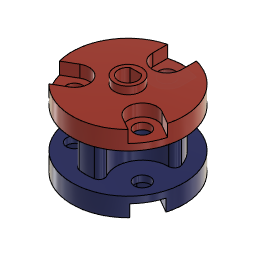
Rotor (Autodesk Fusion 360 design; units mm, degrees)
Autodesk Fusion 360 part; units mm, degrees
sketch "Sketch1" plane through (0, 0, 0) normal (0, 0, 1) x (1, 0, 0)
  circle A0 centre (0, 0) radius 15
  dimension "d1" = 30
  constraint coincident A0.centre origin
  measures "d1" diameter of A0
extrude "Extrude1" add sketch "Sketch1" along normal blind 5 contours A0 picked at (3.831549, 5.619851) makes body 1
sketch "Sketch2" plane through (0, 0, 5) normal (0, 0, 1) x (-1, 0, 0)
  circle A0 centre (0, 0) radius 15
  circle A1 centre (0, 0) radius 2.6
  circle A2 centre (0, 0) radius 3.6
  line L0 (0.004273, -1.599996) -> (2.049393, -1.599996)
  line L1 (0.004273, -1.599996) -> (-2.049393, -1.599996)
  dimension "d4" = 5.2
  dimension "d5" = 1
  constraint concentric A0 A1
  measures "d4" diameter of A1
extrude "Extrude2" add sketch "Sketch2" along normal blind 2 contours A2 picked at (-3.178319, -0.724982) bodies 1
extrude "Extrude3" cut 1 faces at (-0.716074, -0.488211, 5) along direction (0, 0, -1) blind 5 on bodies 1 bodies 1
sketch "Sketch3" plane through (0, 0, 5) normal (0, 0, 1) x (-1, 0, 0)
  circle A0 centre (0, 0) radius 15
  circle A1 centre (0, 0) radius 3.6
  arc A2 (0, -15) -> (12.990381, 7.5) centre (0, 0) ccw
  line L0 (0, 0) -> (0, -15) construction
  line L1 (0, 0) -> (12.990381, 7.5) construction
  arc A3 (-12.990381, 7.5) -> (0, -15) centre (0, 0) ccw
  line L2 (0, 0) -> (-12.990381, 7.5) construction
  line L3 (0, 0) -> (0, -15) construction
  circle A4 centre (0, -11.5) radius 3.5
  circle A5 centre (-9.959292, 5.75) radius 3.5
  line L4 (0, -11.5) -> (3.5, -11.5)
  line L5 (-3.5, -11.498985) -> (0.073703, -11.498985)
  line L6 (3.5, -11.5) -> (3.5, -14.585952)
  line L7 (-3.5, -11.5) -> (-3.5, -14.585952)
  line L8 (3.5, -11.5) -> (0, -8)
  line L9 (-3.5, -11.498985) -> (0, -8)
  arc A6 (0, -15) -> (12.990381, -7.5) centre (0, 0) ccw
  line L10 (0, 0) -> (0, -15) construction
  line L11 (0, 0) -> (12.990381, -7.5) construction
  line L12 (0, 0) -> (0, 15)
  line L13 (-8.209292, 8.781089) -> (-10.881805, 10.324065)
  circle A7 centre (-9.959292, 5.75) radius 3.5
  line L14 (-8.208413, 8.780581) -> (-9.995265, 5.685663)
  line L15 (-8.208413, 8.780581) -> (-6.928203, 4)
  line L16 (-11.709292, 2.718911) -> (-6.928203, 4)
  line L17 (-9.959292, 5.75) -> (-11.709292, 2.718911)
  line L18 (-11.709292, 2.718911) -> (-14.381805, 4.261887)
  circle A8 centre (9.959292, 5.75) radius 3.5
  line L19 (11.709292, 2.718911) -> (14.381805, 4.261887)
  line L20 (9.959292, 5.75) -> (11.709292, 2.718911)
  line L21 (11.709292, 2.718911) -> (6.928203, 4)
  line L22 (8.208413, 8.780581) -> (6.928203, 4)
  line L23 (8.208413, 8.780581) -> (9.995265, 5.685663)
  line L24 (8.209292, 8.781089) -> (10.881805, 10.324065)
  circle A9 centre (9.959292, 5.75) radius 2.25
  circle A10 centre (-9.959292, 5.75) radius 2.25
  circle A11 centre (0, -11.5) radius 2.25
  point P0 (0, -15)
  dimension "d10" = 120
  dimension "d11" = 120
  dimension "d12" = 7
  dimension "d14" = 7
  dimension "d15" = 60
  dimension "d18" = 4.5
  dimension "d19" = 4.5
  dimension "d20" = 4.5
  constraint coincident A0 P0
  constraint coincident P0 A2.start
  constraint coincident A0.centre A1.centre
  constraint coincident P0 A4
  constraint coincident A4.centre L4.start
  constraint coincident A4 L4.end
  constraint perpendicular L3 L4
  constraint horizontal L5
  constraint perpendicular L0 L5
  constraint vertical L6
  constraint symmetric L0 L4.end L7.start
  constraint coincident L3 L8.end
  constraint coincident A4 L8.end
  constraint coincident A0 L12.end
  constraint vertical L12
  constraint symmetric A5 L12 A8
  constraint concentric A5 A10
  measures "d10" angle of L0 L1
  measures "d11" angle of L2 L3
  measures "d12" diameter of A4
  measures "d14" diameter of A5
  measures "d15" angle of L10 L11
  measures "d18" diameter of A9
  measures "d19" diameter of A10
  measures "d20" diameter of A11
extrude "Extrude4" cut sketch "Sketch3" against normal blind 2 contours A0 A2 A8 L19 | A0 A8 L24 | A8 L20 L23 A9 | L20 L21 L22 L23 A9 | A8 L21 | A0 A2 A4 L6 A6 | A8 L22 | L20 L23 A9 | L20 L23 A9 | A0 A3 A4 L7 | A4 L4 L5 A11 | A4 L8 | L4 L5 L8 L9 A11 | A4 L9 | L4 L5 A11 | L4 L5 A11 | A0 A5 L13 A7 | A0 A3 A5 A7 L18 | A5 A7 L14 L17 A10 | L14 L15 L16 L17 A10 | A5 A7 L15 | A5 A7 L16 | L14 L17 A10 | L14 L17 A10 picked at (13.896299, 4.785613) picked at (11.214438, 9.606876) picked at (13.021218, 5.464336) picked at (7.653691, 4.418471) picked at (8.615201, 3.435118) picked at (2.712464, -14.515527) picked at (7.199952, 6.23225) picked at (8.941426, 6.846078) picked at (10.607678, 7.09766) picked at (-2.71258, -14.515426) picked at (-0.222289, -14.569344) picked at (1.883413, -9.122938) picked at (0.000337, -8.837526) picked at (-2.084639, -9.297057) picked at (-1.458441, -11.832237) picked at (-1.491575, -11.387223) picked at (-11.214583, 9.606826) picked at (-13.927047, 4.908701) picked at (-12.728453, 7.092403) picked at (-7.653523, 4.418764) picked at (-7.238682, 5.875074) picked at (-9.965869, 3.073208) picked at (-8.467382, 5.638053) picked at (-10.399735, 7.179237) bodies 1
extrude "Extrude5" cut sketch "Sketch3" against normal blind 5 contours L20 L23 A9 | L20 L23 A9 | L4 L5 A11 | L4 L5 A11 | L14 L17 A10 | L14 L17 A10 picked at (8.941426, 6.846078) picked at (10.607678, 7.09766) picked at (-1.458441, -11.832237) picked at (-1.491575, -11.387223) picked at (-8.467382, 5.638053) picked at (-10.399735, 7.179237) bodies 1
extrude "Extrude6" add sketch "Sketch2" against normal blind 5 contours A1 L0 L1 picked at (0.001424, -2.26244) bodies 1
extrude "Extrude7" add 1 faces at (0.602223, 1.689912, 5) along direction (0, 0, 1) blind 2 on bodies 1 bodies 1
sketch "Sketch4" plane through (0, 0, 0) normal (0, 0, -1) x (1, 0, 0)
  circle A0 centre (0, -11.5) radius 2.25
  circle A1 centre (9.959292, 5.75) radius 2.25
  circle A2 centre (-9.959292, 5.75) radius 2.25
  arc A3 (2.049393, -1.599996) -> (-2.049393, -1.599996) centre (0, 0) ccw
  line L0 (2.049393, -1.599996) -> (-2.049393, -1.599996)
  circle A4 centre (0, 0) radius 15
extrude "Extrude8" add sketch "Sketch4" against normal blind 7 contours A3 L0 picked at (0.587293, -0.429327) bodies 1
sketch "Sketch5" plane through (0, 0, 7) normal (0, 0, 1) x (-1, 0, 0)
  circle A0 centre (0, 0) radius 3.6
  circle A1 centre (0, 0) radius 2.575
  line L0 (0, 0) -> (0, 2.575)
  line L1 (0, 2.575) -> (0, -2.075)
  line L2 (0, -2.075) -> (7, -2.075)
  line L3 (7, -2.075) -> (0, -2.075)
  line L4 (-5.579458, -2.075) -> (0, -2.075)
  dimension "d30" = 5.15
  dimension "d31" = 4.65
  constraint concentric A0 A1
  constraint coincident A0.centre A1.centre
  constraint coincident A1 L0.end
  constraint vertical L0
  constraint parallel L0 L1
  constraint perpendicular L1 L2
  constraint perpendicular L1 L4
  measures "d30" diameter of A1
  measures "d31" distance of L0.end L1.end
extrude "Extrude9" cut sketch "Sketch5" against normal blind 7 contours A1 L0 L1 L4 | A1 L0 L1 L2 L3 picked at (-0.508265, -1.383333) picked at (0.508265, -1.383333) bodies 1
sketch "Sketch6" plane through (0, 0, 0) normal (0, 0, -1) x (1, 0, 0)
  line L0 (1.524795, -2.075) -> (-1.524795, -2.075)
  arc A0 (1.524795, -2.075) -> (-1.524795, -2.075) centre (0, 0) ccw
  circle A1 centre (0, -11.5) radius 2.25
  circle A2 centre (9.959292, 5.75) radius 2.25
  circle A3 centre (-9.959292, 5.75) radius 2.25
  circle A4 centre (0, 0) radius 15
  circle A5 centre (0, 0) radius 2.575
  circle A6 centre (0, 0) radius 3.575
  dimension "d34" = 1
  constraint coincident A0.centre A4.centre
extrude "Extrude10" add sketch "Sketch6" along normal blind 10 separate body contours L0 A5 | L0 A0 A5 | A6 picked at (0.406148, -2.139494) picked at (-0.543001, 0.409482) picked at (-3.0114, 1.181824) makes body 2
sketch "Sketch7" plane through (0, 0, -10) normal (0, 0, -1) x (1, 0, 0)
  circle A0 centre (0, 0) radius 3.575
  circle A1 centre (0, 0) radius 15
  dimension "d37" = 30
  constraint coincident A0.centre A1.centre
  measures "d37" diameter of A1
extrude "Extrude11" add sketch "Sketch7" along normal blind 5 contours A0 | A1 picked at (-1.243849, -0.464547) picked at (11.122511, -0.92282) bodies 2
sketch "Sketch8" plane through (0, 0, 0) normal (0, 0, -1) x (1, 0, 0)
  line L0 (1.524795, -2.075) -> (-1.524795, -2.075)
  arc A0 (1.524795, -2.075) -> (-1.524795, -2.075) centre (0, 0) ccw
  circle A1 centre (0, -11.5) radius 2.25
  circle A2 centre (9.959292, 5.75) radius 2.25
  circle A3 centre (-9.959292, 5.75) radius 2.25
  circle A4 centre (0, 0) radius 15
extrude "Extrude12" cut sketch "Sketch8" along normal blind 22 contours A1 | A2 | A3 picked at (0.642406, -11.395654) picked at (10.453033, 5.512227) picked at (-11.028245, 5.848384) bodies 2
sketch "Sketch9" plane through (0, 0, -15) normal (0, 0, -1) x (1, 0, 0)
  circle A0 centre (9.959292, 5.75) radius 2.25
  circle A1 centre (-9.959292, 5.75) radius 2.25
  circle A2 centre (0, -11.5) radius 2.25
  circle A3 centre (0, 0) radius 15
  circle A4 centre (0, -11.5) radius 3.5
  line L0 (-3.491404, -11.74515) -> (-3.491404, -14.588012)
  line L1 (3.491404, -11.74515) -> (3.491404, -14.588012)
  dimension "d42" = 1.25
  constraint vertical L0
extrude "Extrude13" cut sketch "Sketch9" against normal blind 2 contours A3 A4 L0 | A3 A4 L1 | A4 picked at (-2.795512, -14.431964) picked at (2.795512, -14.431964) picked at (-3.043001, -11.043038) bodies 2
sketch "Sketch10" plane through (0, 0, -15) normal (0, 0, -1) x (1, 0, 0)
  line L0 (3.491404, -11.74515) -> (3.491404, -14.588012)
  arc A0 (3.491404, -14.588012) -> (-3.491404, -14.588012) centre (0, 0) ccw
  line L1 (-3.491404, -14.588012) -> (-3.491404, -11.74515)
  arc A1 (3.491404, -11.74515) -> (-3.491404, -11.74515) centre (0, -11.5) ccw
  circle A2 centre (9.959292, 5.75) radius 2.25
  circle A3 centre (-9.959292, 5.75) radius 2.25
  circle A4 centre (9.959292, 5.75) radius 3.5
  line L2 (11.462802, 2.589389) -> (14.453488, 4.012066)
  line L3 (7.973878, 8.632383) -> (10.701295, 10.511055)
  dimension "d45" = 1.25
  constraint tangent A4 L2
extrude "Extrude14" cut sketch "Sketch10" against normal blind 2 contours A0 A4 L2 | A0 A4 L3 | A4 picked at (13.946432, 4.667869) picked at (10.993121, 9.749366) picked at (7.187387, 4.414504) bodies 2
sketch "Sketch11" plane through (0, 0, -15) normal (0, 0, -1) x (1, 0, 0)
  line L0 (7.973878, 8.632383) -> (10.701295, 10.511055)
  arc A0 (10.701295, 10.511055) -> (-3.491404, -14.588012) centre (0, 0) ccw
  line L1 (-3.491404, -14.588012) -> (-3.491404, -11.74515)
  arc A1 (3.491404, -11.74515) -> (-3.491404, -11.74515) centre (0, -11.5) ccw
  line L2 (3.491404, -11.74515) -> (3.491404, -14.588012)
  arc A2 (3.491404, -14.588012) -> (14.453488, 4.012066) centre (0, 0) ccw
  line L3 (14.453488, 4.012066) -> (11.462802, 2.589389)
  arc A3 (7.973878, 8.632383) -> (11.462802, 2.589389) centre (9.959292, 5.75) ccw
  circle A4 centre (-9.959292, 5.75) radius 2.25
  circle A5 centre (-9.959292, 5.75) radius 3.5
  line L4 (-8.338485, 8.852093) -> (-10.972053, 10.228102)
  line L5 (-9.959292, 5.75) -> (-11.907849, 6.875)
  line L6 (-11.83538, 2.795293) -> (-14.343822, 4.388025)
  dimension "d48" = 1.25
  constraint tangent A5 L4
extrude "Extrude15" cut sketch "Sketch11" against normal blind 2 contours A0 A5 L4 | A0 A5 L6 | A5 picked at (-11.284058, 9.544525) picked at (-13.90783, 5.000018) picked at (-11.411346, 3.036744) bodies 2
sketch "Sketch12" plane through (0, 0, 7) normal (0, 0, 1) x (-1, 0, 0)
  line L0 (1.524795, -2.075) -> (-1.524795, -2.075)
  arc A0 (1.524795, -2.075) -> (-1.524795, -2.075) centre (0, 0) ccw
  circle A1 centre (0, 0) radius 3.6
extrude "Extrude16" cut sketch "Sketch12" against normal blind 22 contours L0 A0 picked at (0.664347, -0.839845) bodies 2
sketch "Sketch13" plane through (0, 0, -15) normal (0, 0, -1) x (1, 0, 0)
  line L0 (1.524795, -2.075) -> (-1.524795, -2.075)
  arc A0 (1.524795, -2.075) -> (-1.524795, -2.075) centre (0, 0) ccw
  line L1 (-10.972053, 10.228102) -> (-8.338485, 8.852093)
  arc A1 (-11.83538, 2.795293) -> (-8.338485, 8.852093) centre (-9.959292, 5.75) ccw
  line L2 (-11.83538, 2.795293) -> (-14.343822, 4.388025)
  arc A2 (-14.343822, 4.388025) -> (-3.491404, -14.588012) centre (0, 0) ccw
  line L3 (-3.491404, -14.588012) -> (-3.491404, -11.74515)
  arc A3 (3.491404, -11.74515) -> (-3.491404, -11.74515) centre (0, -11.5) ccw
  line L4 (3.491404, -11.74515) -> (3.491404, -14.588012)
  arc A4 (3.491404, -14.588012) -> (14.453488, 4.012066) centre (0, 0) ccw
  line L5 (14.453488, 4.012066) -> (11.462802, 2.589389)
  arc A5 (7.973878, 8.632383) -> (11.462802, 2.589389) centre (9.959292, 5.75) ccw
  line L6 (7.973878, 8.632383) -> (10.701295, 10.511055)
  arc A6 (10.701295, 10.511055) -> (-10.972053, 10.228102) centre (0, 0) ccw
  circle A7 centre (0, 0) radius 2.575
  circle A8 centre (0, 0) radius 4.075
  dimension "d53" = 1.5
  constraint concentric A0 A7
extrude "Extrude17" add sketch "Sketch13" along normal blind 1.5 contours A8 picked at (-3.320824, 1.303264) bodies 2
extrude "Extrude18" cut 1 faces at (0.406148, 2.139494, -15) along direction (0, 0, 1) blind 2.5 on bodies 2 bodies 2
extrude "Extrude19" add 3 faces at (-3.003329, 12.936467, -13) (9.377931, -9.029009, -13) (-12.665844, -3.888616, -13) along direction (0, 0, -1) blind 2 on bodies 2 bodies 2
sketch "Sketch14" plane through (0, 0, 0) normal (0, 0, -1) x (1, 0, 0)
  line L0 (1.524795, -2.075) -> (-1.524795, -2.075)
  arc A0 (1.524795, -2.075) -> (-1.524795, -2.075) centre (0, 0) ccw
  circle A1 centre (0, -11.5) radius 2.25
  circle A2 centre (9.959292, 5.75) radius 2.25
  circle A3 centre (-9.959292, 5.75) radius 2.25
  circle A4 centre (0, 0) radius 15
extrude "Extrude20" add sketch "Sketch14" against normal blind 3 contours A1 | A2 | A3 picked at (0.642406, -11.395654) picked at (10.453033, 5.512227) picked at (-11.028245, 5.848384) bodies 1
extrude "Extrude21" add 3 faces at (0, 12.666328, 3) (-10.438211, -4.978905, 3) (10.969655, -6.333333, 3) along direction (0, 0, 1) blind 2 on bodies 1 bodies 1
sketch "Sketch15" plane through (0, 0, -15) normal (0, 0, -1) x (1, 0, 0)
  circle A0 centre (-9.959292, 5.75) radius 2.25
  circle A1 centre (0, -11.5) radius 2.25
  circle A2 centre (9.959292, 5.75) radius 2.25
  circle A3 centre (0, 0) radius 15
  circle A4 centre (0, 0) radius 4.075
extrude "Extrude22" add sketch "Sketch15" against normal blind 5 contours A0 | A1 | A2 picked at (-11.028245, 5.848384) picked at (0.642406, -11.395654) picked at (10.383143, 5.424587) bodies 2
extrude "Extrude23" add 1 faces at (-3.320824, -1.303264, -16.5) along direction (0, 0, -1) blind 0.5 on bodies 2 bodies 2
sketch "Sketch16" plane through (0, 0, 5) normal (0, 0, 1) x (-1, 0, 0)
  circle A0 centre (0, 0) radius 3.6
  circle A1 centre (0, 0) radius 15
  line L0 (0, -15) -> (0, -10.5)
  circle A2 centre (0, -10.5) radius 2.125
  circle A3 centre (0, -10.5) radius 3.875
  line L1 (0, -10.5) -> (-3.875, -10.5)
  line L2 (-3.875, -10.5) -> (-3.875, -14.490838)
  line L3 (0, -10.5) -> (3.875, -10.5)
  line L4 (3.875, -10.5) -> (3.875, -14.490838)
  circle A4 centre (9.093267, 5.25) radius 3.875
  circle A5 centre (9.093267, 5.25) radius 2.125
  line L5 (11.030767, 1.894152) -> (14.486934, 3.88957)
  line L6 (9.093267, 5.25) -> (11.030767, 1.894152)
  line L7 (9.093267, 5.25) -> (7.155767, 8.605848)
  line L8 (7.155767, 8.605848) -> (10.611934, 10.601267)
  line L9 (12.990381, 7.5) -> (9.093267, 5.25)
  circle A6 centre (-9.093267, 5.25) radius 3.875
  circle A7 centre (-9.093267, 5.25) radius 2.125
  line L10 (-7.155767, 8.605848) -> (-10.611934, 10.601267)
  line L11 (-9.093267, 5.25) -> (-7.155767, 8.605848)
  line L12 (-9.093267, 5.25) -> (-11.030767, 1.894152)
  line L13 (-11.030767, 1.894152) -> (-14.486934, 3.88957)
  line L14 (-12.990381, 7.5) -> (-9.093267, 5.25)
  dimension "d68" = 4.5
  dimension "d69" = 4.25
  dimension "d70" = 7.75
  dimension "d72" = 360
  constraint coincident A1 L0.start
  constraint vertical L0
  constraint coincident L0.end A2.centre
  constraint coincident A3 L1.end
  constraint perpendicular L0 L1
  constraint tangent A3 L2
  constraint coincident A3 L3.end
  constraint perpendicular L0 L3
  constraint tangent A3 L4
  measures "d68" distance of L0.start L0.end
  measures "d69" diameter of A2
  measures "d70" diameter of A3
extrude "Extrude24" cut sketch "Sketch16" against normal blind 3.25 contours A1 A4 L5 L9 | A1 L0 A3 L4 | A1 A4 L8 L9 | A4 A5 L6 L9 | A4 A5 L6 L7 | A1 L0 A3 L2 | A2 A3 L1 L3 | L0 A2 A3 L3 | A4 A5 L7 L9 | L0 A2 A3 L1 | A1 A6 L10 L14 | A1 A6 L13 L14 | A6 A7 L11 L14 | A6 A7 L11 L12 | A6 A7 L12 L14 picked at (13.835196, 4.565686) picked at (3.004119, -14.230785) picked at (10.822162, 9.717036) picked at (12.362595, 4.951915) picked at (10.565166, 2.315571) picked at (-3.004119, -14.230785) picked at (2.816229, -8.812927) picked at (2.357361, -12.785898) picked at (8.964615, 8.531147) picked at (-0.183823, -13.778519) picked at (-10.822162, 9.717036) picked at (-13.826281, 4.51375) picked at (-11.783989, 7.132151) picked at (-5.816027, 5.057487) picked at (-10.975418, 2.559278) bodies 1
extrude "Extrude25" cut 3 faces at (8.757496, -4.696203, 5) (-1.276122, 10.845562, 5) (-9.630289, -4.650268, 5) along direction (0, 0, -1) blind 39 on bodies 1 bodies 1 2
sketch "Sketch17" plane through (0, 0, -15) normal (0, 0, -1) x (1, 0, 0)
  circle A0 centre (0, -10.5) radius 2.125
  circle A1 centre (9.093267, 5.25) radius 2.125
  circle A2 centre (-9.093267, 5.25) radius 2.125
  circle A3 centre (0, 0) radius 15
  circle A4 centre (0, 0) radius 4.075
  line L0 (3.55, -8.450407) -> (0, -6.400813)
  line L1 (0, -6.400813) -> (-3.55, -8.450407)
  line L2 (-3.55, -8.450407) -> (-3.55, -12.549593)
  line L3 (-3.55, -12.549593) -> (0, -14.599187)
  line L4 (0, -14.599187) -> (3.55, -12.549593)
  line L5 (3.55, -12.549593) -> (3.55, -8.450407)
  line L6 (-3.55, -12.549593) -> (-3.55, -14.573864)
  line L7 (3.55, -12.549593) -> (3.55, -14.573864)
  line L8 (12.643267, 3.200407) -> (14.396336, 4.212542)
  line L9 (9.093267, 1.150813) -> (12.643267, 3.200407)
  line L10 (5.543267, 3.200407) -> (9.093267, 1.150813)
  line L11 (5.543267, 7.299593) -> (5.543267, 3.200407)
  line L12 (9.093267, 9.349187) -> (5.543267, 7.299593)
  line L13 (9.093267, 9.349187) -> (10.846336, 10.361322)
  line L14 (12.643267, 7.299593) -> (9.093267, 9.349187)
  line L15 (12.643267, 3.200407) -> (12.643267, 7.299593)
  line L16 (-9.093267, 9.349187) -> (-10.846336, 10.361322)
  line L17 (-5.543267, 7.299593) -> (-9.093267, 9.349187)
  line L18 (-5.543267, 3.200407) -> (-5.543267, 7.299593)
  line L19 (-9.093267, 1.150813) -> (-5.543267, 3.200407)
  line L20 (-12.643267, 3.200407) -> (-9.093267, 1.150813)
  line L21 (-12.643267, 3.200407) -> (-14.396336, 4.212542)
  line L22 (-12.643267, 7.299593) -> (-12.643267, 3.200407)
  line L23 (-9.093267, 9.349187) -> (-12.643267, 7.299593)
  point P0 (0, -10.5)
  dimension "d77" = 3.55
  dimension "d79" = 360
  constraint coincident P0 A0.centre
  constraint parallel L2 L6
  constraint parallel L5 L7
  measures "d77" distance of P0 L5
extrude "Extrude26" cut sketch "Sketch17" against normal blind 3.25 contours A3 L8 L13 L14 L15 | A3 L3 L4 L6 L7 | L9 L10 L11 L12 L14 L15 | L0 L1 L2 L3 L4 L5 | A3 L16 L21 L22 L23 | L17 L18 L19 L20 L22 L23 picked at (13.026065, 5.466104) picked at (-1.779247, -14.013955) picked at (10.630767, 2.586972) picked at (-1.5375, -7.836972) picked at (-11.246817, 8.547851) picked at (-7.555767, 7.913028) bodies 2
sketch "Sketch18" plane through (0, 0, -10) normal (0, 0, 1) x (-1, 0, 0)
  circle A0 centre (0, -10.5) radius 2.125
  circle A1 centre (-9.093267, 5.25) radius 2.125
  circle A2 centre (9.093267, 5.25) radius 2.125
  circle A3 centre (0, 0) radius 15
  circle A4 centre (0, 0) radius 3.575
extrude "Extrude27" add sketch "Sketch18" along normal blind 10 contours A3 picked at (8.894743, -0.781378) bodies 2
sketch "Sketch19" plane through (0, 0, 0) normal (0, 0, 1) x (-1, 0, 0)
  circle A0 centre (0, 0) radius 15
  circle A1 centre (0, -10.5) radius 2.125
  circle A2 centre (-9.093267, 5.25) radius 2.125
  circle A3 centre (9.093267, 5.25) radius 2.125
  line L0 (1.524795, -2.075) -> (-1.524795, -2.075)
  arc A4 (1.524795, -2.075) -> (-1.524795, -2.075) centre (0, 0) ccw
  circle A5 centre (9.093267, 5.25) radius 7
  circle A6 centre (-9.093267, 5.25) radius 7
  circle A7 centre (0, -10.5) radius 7
  dimension "d84" = 14
  dimension "d85" = 14
  dimension "d86" = 14
  constraint concentric A3 A5
  constraint concentric A2 A6
  constraint concentric A1 A7
  measures "d84" diameter of A5
  measures "d85" diameter of A6
  measures "d86" diameter of A7
extrude "Extrude28" cut sketch "Sketch19" against normal blind 10 contours A0 A5 | A0 A7 | A0 A6 picked at (8.874277, 10.098602) picked at (-4.307696, -12.73711) picked at (-13.187756, 2.641635) bodies 2
fillet "Fillet1" radius 2.5 6 edges at (-14.935132, -1.393498, -5) (-8.67437, -12.237455, -5) (6.260762, 13.630952, -5) (-6.260762, 13.630952, -5) (8.67437, -12.237455, -5) (14.935132, -1.393498, -5) on bodies 2
extrude "Extrude29" add 4 faces at (9.261833, 5.756006, 0) (-0.066096, 2.550936, 0) (-9.615764, 5.14298, 0) (-0.353931, -10.898986, 0) along direction (0, 0, 1) blind 2 on bodies 2 bodies 2
sketch "Sketch20" plane through (0, 0, 1.75) normal (0, 0, 1) x (-1, 0, 0)
  circle A0 centre (0, -10.5) radius 2.125
  line L0 (-3.875, -10.5) -> (-3.875, -14.490838)
  arc A1 (-3.875, -14.490838) -> (3.875, -14.490838) centre (0, 0) ccw
  line L1 (3.875, -14.490838) -> (3.875, -10.5)
  arc A2 (3.875, -10.5) -> (-3.875, -10.5) centre (0, -10.5) ccw
move_body "Move1" bodies 1 to x (1, 0, 0) y (0, 1, 0) z (0, 0, 1) at (0, 0, 2)
extrude "Extrude30" cut 1 faces at (-9.615764, 5.14298, 2) along direction (0, 0, -1) blind 1.5 on bodies 2 bodies 2
move_body "Move2" bodies 1 to x (1, 0, 0) y (0, 1, 0) z (0, 0, 1) at (0, 0, -1.5)
copy_body "CopyPasteBodies1" bodies 2 makes body 3
sketch "Sketch21" plane through (0, 0, 0.5) normal (0, 0, 1) x (-1, 0, 0)
  line L0 (1.524795, -2.075) -> (-1.524795, -2.075)
  arc A0 (1.524795, -2.075) -> (-1.524795, -2.075) centre (0, 0) ccw
  arc A1 (-11.161467, -1.437492) -> (-14.280133, -4.591058) centre (-11.90011, -3.825882) ccw
  arc A2 (-14.280133, -4.591058) -> (-11.116039, -10.071429) centre (0, 0) ccw
  arc A3 (-11.116039, -10.071429) -> (-6.825638, -8.947368) centre (-9.263366, -8.392857) ccw
  arc A4 (6.825638, -8.947368) -> (-6.825638, -8.947368) centre (0, -10.5) ccw
  arc A5 (6.825638, -8.947368) -> (11.116039, -10.071429) centre (9.263366, -8.392857) ccw
  arc A6 (11.116039, -10.071429) -> (14.280133, -4.591058) centre (0, 0) ccw
  arc A7 (14.280133, -4.591058) -> (11.161467, -1.437492) centre (11.90011, -3.825882) ccw
  arc A8 (4.335829, 10.38486) -> (11.161467, -1.437492) centre (9.093267, 5.25) ccw
  arc A9 (4.335829, 10.38486) -> (3.164093, 14.662487) centre (2.636745, 12.218739) ccw
  arc A10 (3.164093, 14.662487) -> (-3.164093, 14.662487) centre (0, 0) ccw
  arc A11 (-3.164093, 14.662487) -> (-4.335829, 10.38486) centre (-2.636745, 12.218739) ccw
  arc A12 (-11.161467, -1.437492) -> (-4.335829, 10.38486) centre (-9.093267, 5.25) ccw
  circle A13 centre (0, 0) radius 11.253654
  constraint concentric A0 A13
sketch "Sketch28" plane through (0, 0, 0.5) normal (0, 0, 1) x (-1, 0, 0)
  line L0 (1.524795, -2.075) -> (-1.524795, -2.075)
  arc A0 (1.524795, -2.075) -> (-1.524795, -2.075) centre (0, 0) ccw
  arc A1 (-11.161467, -1.437492) -> (-14.280133, -4.591058) centre (-11.90011, -3.825882) ccw
  arc A2 (-14.280133, -4.591058) -> (-11.116039, -10.071429) centre (0, 0) ccw
  arc A3 (-11.116039, -10.071429) -> (-6.825638, -8.947368) centre (-9.263366, -8.392857) ccw
  arc A4 (6.825638, -8.947368) -> (-6.825638, -8.947368) centre (0, -10.5) ccw
  arc A5 (6.825638, -8.947368) -> (11.116039, -10.071429) centre (9.263366, -8.392857) ccw
  arc A6 (11.116039, -10.071429) -> (14.280133, -4.591058) centre (0, 0) ccw
  arc A7 (14.280133, -4.591058) -> (11.161467, -1.437492) centre (11.90011, -3.825882) ccw
  arc A8 (4.335829, 10.38486) -> (11.161467, -1.437492) centre (9.093267, 5.25) ccw
  arc A9 (4.335829, 10.38486) -> (3.164093, 14.662487) centre (2.636745, 12.218739) ccw
  arc A10 (3.164093, 14.662487) -> (-3.164093, 14.662487) centre (0, 0) ccw
  arc A11 (-3.164093, 14.662487) -> (-4.335829, 10.38486) centre (-2.636745, 12.218739) ccw
  arc A12 (-11.161467, -1.437492) -> (-4.335829, 10.38486) centre (-9.093267, 5.25) ccw
  circle A13 centre (0, 0) radius 11.253654
  constraint coincident A0.centre A2.centre
extrude "Extrude38" cut sketch "Sketch28" against normal blind 10.5 contours A1 A2 A3 A13 | A9 A10 A11 A13 | A5 A6 A7 A13 picked at (-11.88718, -6.863067) picked at (0, 13.726133) picked at (11.88718, -6.863067) bodies 2
fillet "Fillet3" radius 1.5 6 edges at (4.335829, -10.38486, -4.75) (-4.335829, -10.38486, -4.75) (-11.161467, 1.437492, -4.75) (-6.825638, 8.947368, -4.75) (6.825638, 8.947368, -4.75) (11.161467, 1.437492, -4.75) on bodies 2
extrude "Extrude39" [rolled back] along distance -10.5 taper angle 0
hidden bodies 3
equation "d56 = 1.50 mm - 4 mm"
